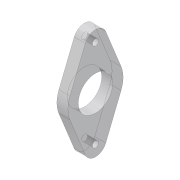
# Autodesk Inventor part: M14 - Upper Bearing Support
Saved by Autodesk Inventor 2016 (Build 200138000, 138)
## iProperties
Created: 2016-12-26
Part Number: M14 - Upper Bearing Support
Material: Polycarbonate, Clear
Document SubType Name: Modeling
Designer: Fernando
Stock Number: 0
Mass: 15.3401 g
Surface Area: 55.4936 cm^2
Volume: 12.7834 cm^3
Density: 1.2 g/cm^3
Appearance: Polycarbonate - Clear
SurfaceArea_m2: .01
Author: Fernando
Autodesk Inventor part; units mm, degrees
ref_plane "YZ Plane" through (0, 0, 0) normal (1, 0, 0) x (0, 1, 0)
ref_plane "XZ Plane" through (0, 0, 0) normal (0, 1, 0) x (-1, 0, 0)
ref_plane "XY Plane" through (0, 0, 0) normal (0, 0, 1) x (1, 0, 0)
sketch "Sketch4" plane through (0, 0, 0) normal (1, 0, 0) x (0, 1, 0)
  circle A0 centre (0, 0) radius 12.5
  arc A1 (-7.4162, -35) -> (7.4162, -35) centre (0, -32) ccw
  arc A2 (7.4162, 35) -> (-7.4162, 35) centre (0, 32) ccw
  line L0 (7.4162, 35) -> (18.5405, 7.5)
  line L1 (-7.4162, 35) -> (-18.5405, 7.5)
  line L2 (-18.5405, -7.5) -> (-7.4162, -35)
  line L3 (7.4162, -35) -> (18.5405, -7.5)
  arc A3 (-18.5405, 7.5) -> (-18.5405, -7.5) centre (0, 0) ccw
  arc A4 (18.5405, -7.5) -> (18.5405, 7.5) centre (0, 0) ccw
  circle A5 centre (0, 32) radius 2.25
  circle A6 centre (0, -32) radius 2.25
  line L4 (0, 32) -> (0, 0) construction
  line L5 (0, 0) -> (0, -32) construction
  dimension "d32" = 4.5
  dimension "d33" = 4.5
  dimension "d34" = 25
  dimension "d35" = 8
  dimension "d36" = 64
  dimension "d37" = 20
  constraints: 12 end point, 8 point on circle, 8 tangent, 7 centre point, 5 coincident, 2 parallel, 2 vertical, 1 collinear
  measures "d32" diameter of A6
  measures "d33" diameter of A5
  measures "d34" diameter of A0
  measures "d35" radius of A2
  measures "d36" distance of A6.centre L4.start
  measures "d37" radius of A4
extrude "Extrusion2" add sketch "Sketch4" along normal blind 8
body "Solid3"
